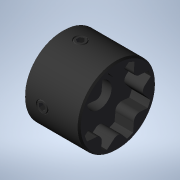
# Autodesk Inventor part: MSF-25 - 6-8 Casing 2
Saved by Autodesk Inventor 2021 (Build 250183000, 183)
## iProperties
Created: 2026-05-20
Part Number: MSF-25 - 6-8 Casing 2
Material: Generic
Catalog Web Link: www.3dfindit.com
Description: MSF right-MSF
Vendor: NBK
Document SubType Name: Modeling
Designer: psAdmin
Manufacturer: NBK
Mass: 6.39983 g
Surface Area: 31.7975 cm^2
Volume: 6.39983 cm^3
Density: 1 g/cm^3
Appearance: PSOLRGB-176-176-176
Category: PARTsolutions
Company: NBK
Title: MSF-25
Author: Cadenas PARTsolutions
Comments: MSF
PSOL_IDENT_0: {$CADENAS_DATA/23d-libs/nbk/motion_control_parts/couplicon_mini/msf/msf_right.prj},174 {VTYP=3D},{NB=
PSOL_IDENT_1: MSF-25 - 6-8 Casing 2},{LINA=MSF-25},{NN=MSF right},{DATE=08.05.2026 02:12:20},{GEOMDATE=08.12.2014
PSOL_IDENT_2: 08:17:09},{VERSION=},{LINEID=40},{WBVAR=D1D2},{WBNUMERIC=}  {NB=MSF-25 - 6-8 Casing 2},{LINA=MSF-25}
PSOL_IDENT_3: ,{KT=DUMMY},{CN=MSF-25},{D1D2=6-8},{D1D2X='6-6','6-6.35','6-8','6-10','6-12','6.35-6.35','6.35-8','6
PSOL_IDENT_4: .35-10','6.35-12','8-8','8-10','8-12','10-10','10-12','12-12'},{A=25},{B=18},{L=12},{W=41},{F=6},{M=
PSOL_IDENT_5: M4},{WT=1.7},{C=17},{K=22},{D=10/10},{NDM=4.000},{KDM=3.242222},{P=0.700},{D1=6},{D2=8},{K1=3.760},{
PSOL_IDENT_6: DU=16.250},{BL=6.000},{H=2.000},{T=1.500}
NB: MSF-25 - 6-8 Casing 2
NN: MSF right
NT: MSF
NBSYN: $CN. - $D1D2. Casing 2
LINA: MSF-25
CATALOG: NBK (Nabeya Bi-tech Kaisha
CN: MSF-25
D1D2: 6-8
D1D2X: '6-6','6-6.35','6-8','6-10','6-12','6.35-6.35','6.35-8','6.35-10','6.35-12','8-8','8-10','8-12','10-10','10-12','12-12'
A: 25
B: 18
L: 12
W: 41
F: 6
M: M4
WT: 1.7
C: 17
K: 22
D: 10/10
NDM: 4
P: 0.7
K1: 3.76
DU: 16.25
BL: 6
H: 2
T: 1.5
SUPPLIER: NBK
ARTICLENO: MSF-25 - 6-8 Casing 2
BOMINFO: MSF-25
CREATOR: CADENAS GmbH
Autodesk Inventor part; units mm, degrees
sketch "Sketch_1" plane through (0, 0, 0) normal (0, 0, 1) x (1, 0, 0)
  line L0 (18, 0) -> (0, 0)
  line L1 (0, 0) -> (0, 12)
  line L2 (0, 12) -> (0.5, 12.5)
  line L3 (0.5, 12.5) -> (17.5, 12.5)
  line L4 (17.5, 12.5) -> (18, 12)
  line L5 (18, 12) -> (18, 0)
  line L6 (18, 0) -> (0, 0)
  constraints: 14 end point
revolve "Revolution1" add sketch "Sketch_1" angle 360 about axis through (18, 0, 0) along (1, 0, 0)
sketch "Sketch_2" plane through (12, 0, 0) normal (1, 0, 0) x (0, 0, -1)
  arc A0 (-10.681, -3.0208) -> (-9.9306, -4.9592) centre (0, 0) ccw
  line L0 (-9.9306, -4.9592) -> (-7.1956, -5.1985)
  arc A1 (-5.1985, -7.1956) -> (-7.1956, -5.1985) centre (-7.0746, -7.0746) ccw
  line L1 (-5.1985, -7.1956) -> (-5.4166, -9.6887)
  arc A2 (-5.4166, -9.6887) -> (-3.5153, -10.5287) centre (0, 0) ccw
  line L2 (-3.5153, -10.5287) -> (-1.4122, -8.764)
  arc A3 (1.4122, -8.764) -> (-1.4122, -8.764) centre (0, -10.005) ccw
  line L3 (1.4122, -8.764) -> (3.0208, -10.681)
  arc A4 (3.0208, -10.681) -> (4.9592, -9.9306) centre (0, 0) ccw
  line L4 (4.9592, -9.9306) -> (5.1985, -7.1956)
  arc A5 (7.1956, -5.1985) -> (5.1985, -7.1956) centre (7.0746, -7.0746) ccw
  line L5 (7.1956, -5.1985) -> (9.6887, -5.4166)
  arc A6 (9.6887, -5.4166) -> (10.5287, -3.5153) centre (0, 0) ccw
  line L6 (10.5287, -3.5153) -> (8.764, -1.4122)
  arc A7 (8.764, 1.4122) -> (8.764, -1.4122) centre (10.005, 0) ccw
  line L7 (8.764, 1.4122) -> (10.681, 3.0208)
  arc A8 (10.681, 3.0208) -> (9.9306, 4.9592) centre (0, 0) ccw
  line L8 (9.9306, 4.9592) -> (7.1956, 5.1985)
  arc A9 (5.1985, 7.1956) -> (7.1956, 5.1985) centre (7.0746, 7.0746) ccw
  line L9 (5.1985, 7.1956) -> (5.4166, 9.6887)
  arc A10 (5.4166, 9.6887) -> (3.5153, 10.5287) centre (0, 0) ccw
  line L10 (3.5153, 10.5287) -> (1.4122, 8.764)
  arc A11 (-1.4122, 8.764) -> (1.4122, 8.764) centre (0, 10.005) ccw
  line L11 (-1.4122, 8.764) -> (-3.0208, 10.681)
  arc A12 (-3.0208, 10.681) -> (-4.9592, 9.9306) centre (0, 0) ccw
  line L12 (-4.9592, 9.9306) -> (-5.1985, 7.1956)
  arc A13 (-7.1956, 5.1985) -> (-5.1985, 7.1956) centre (-7.0746, 7.0746) ccw
  line L13 (-7.1956, 5.1985) -> (-9.6887, 5.4166)
  arc A14 (-9.6887, 5.4166) -> (-10.5287, 3.5153) centre (0, 0) ccw
  line L14 (-10.5287, 3.5153) -> (-8.764, 1.4122)
  arc A15 (-8.764, -1.4122) -> (-8.764, 1.4122) centre (-10.005, 0) ccw
  line L15 (-8.764, -1.4122) -> (-10.681, -3.0208)
  constraints: 32 end point, 32 point on circle, 16 centre point
extrude "Extrusion1" cut sketch "Sketch_2" along normal blind 6
sketch "Sketch3" plane through (0, 0, 0) normal (-1, 0, 0) x (0, 0, 1)
  point P0 (0, 0)
hole "Hole1" at (0, 0, 0) direction (1, 0, 0) diameter 8 depth 12
sketch "Sketch_4" plane through (0, 0, 0) normal (0, 0, 1) x (1, 0, 0)
  line L0 (6, 0) -> (6, 12.5)
  line L1 (6, 12.5) -> (8, 12.5)
  line L2 (8, 12.5) -> (7.6211, 12.1211)
  line L3 (7.6211, 12.1211) -> (7.6211, 0.3789)
  line L4 (7.6211, 0.3789) -> (8, 0)
  line L5 (8, 0) -> (6, 0)
  line L6 (6, 0) -> (6, 12.5)
  constraints: 14 end point
revolve "Revolution2" cut sketch "Sketch_4" angle 360 about axis through (6, 0, 0) along (0, -1, 0)
sketch "Sketch_6" plane through (0, 0, 0) normal (0, 1, 0) x (-1, 0, 0)
  line L0 (-6, 12.5) -> (-6, 0)
  line L1 (-6, 0) -> (-8, 0)
  line L2 (-8, 0) -> (-7.6211, 0.3789)
  line L3 (-7.6211, 0.3789) -> (-7.6211, 12.1211)
  line L4 (-7.6211, 12.1211) -> (-8, 12.5)
  line L5 (-8, 12.5) -> (-6, 12.5)
  line L6 (-6, 12.5) -> (-6, 0)
  constraints: 14 end point
revolve "Revolution3" cut sketch "Sketch_6" angle 360 about axis through (6, 0, 12.5) along (0, 0, 1)
sketch "Sketch_5" plane through (0, 0, -12.5) normal (0, 0, 1) x (1, 0, 0)
  line L0 (11.62, 1.98) -> (11.62, -1.98)
  line L1 (11.62, -1.98) -> (11.9897, -1.98)
  arc A0 (11.9897, -1.98) -> (12.3697, -1.8049) centre (11.9897, -1.48) ccw
  line L2 (12.3697, -1.8049) -> (14.58, 0.78)
  line L3 (14.58, 0.78) -> (14.58, -1.98)
  line L4 (14.58, -1.98) -> (15.18, -1.98)
  line L5 (15.18, -1.98) -> (15.18, 1.98)
  line L6 (15.18, 1.98) -> (14.8103, 1.98)
  arc A1 (14.8103, 1.98) -> (14.4303, 1.8049) centre (14.8103, 1.48) ccw
  line L7 (14.4303, 1.8049) -> (12.22, -0.78)
  line L8 (12.22, -0.78) -> (12.22, 1.98)
  line L9 (12.22, 1.98) -> (11.62, 1.98)
  constraints: 20 end point, 4 point on circle, 2 centre point
extrude "Extrusion2" cut sketch "Sketch_5" along normal blind 0.75
sketch "Sketch_8" plane through (0, 0, -12.5) normal (0, 0, 1) x (1, 0, 0)
  arc A0 (7.0058, 0.1329) -> (7.6, -1.98) centre (7.6, -0.84) ccw
  line L0 (7.6, -1.98) -> (10.08, -1.98)
  line L1 (10.08, -1.98) -> (10.08, 1.98)
  line L2 (10.08, 1.98) -> (7.9, 1.98)
  arc A1 (7.9, 1.98) -> (7.0058, 0.1329) centre (7.9, 0.84) ccw
  arc A2 (7.9, 1.38) -> (7.9, 0.3) centre (7.9, 0.84) ccw
  line L3 (7.9, 0.3) -> (9.48, 0.3)
  line L4 (9.48, 0.3) -> (9.48, 1.38)
  line L5 (9.48, 1.38) -> (7.9, 1.38)
  arc A3 (7.6, -0.3) -> (7.6, -1.38) centre (7.6, -0.84) ccw
  line L6 (7.6, -1.38) -> (9.48, -1.38)
  line L7 (9.48, -1.38) -> (9.48, -0.3)
  line L8 (9.48, -0.3) -> (7.6, -0.3)
  constraints: 18 end point, 8 point on circle, 4 centre point
extrude "Extrusion3" cut sketch "Sketch_8" along normal blind 0.75
sketch "Sketch_9" plane through (0, 0, -12.5) normal (0, 0, 1) x (1, 0, 0)
  line L0 (2.32, 1.38) -> (3.9648, 0)
  line L1 (3.9648, 0) -> (2.32, -1.38)
  line L2 (2.32, -1.38) -> (2.32, -1.98)
  line L3 (2.32, -1.98) -> (2.7016, -1.98)
  arc A0 (2.7016, -1.98) -> (3.0873, -1.8397) centre (2.7016, -1.38) ccw
  line L4 (3.0873, -1.8397) -> (4.68, -0.5034)
  line L5 (4.68, -0.5034) -> (4.68, -1.98)
  line L6 (4.68, -1.98) -> (5.28, -1.98)
  line L7 (5.28, -1.98) -> (5.28, 1.98)
  line L8 (5.28, 1.98) -> (4.68, 1.98)
  line L9 (4.68, 1.98) -> (4.68, 0.5034)
  line L10 (4.68, 0.5034) -> (3.0873, 1.8397)
  arc A1 (3.0873, 1.8397) -> (2.7016, 1.98) centre (2.7016, 1.38) ccw
  line L11 (2.7016, 1.98) -> (2.32, 1.98)
  line L12 (2.32, 1.98) -> (2.32, 1.38)
  constraints: 26 end point, 4 point on circle, 2 centre point
extrude "Extrusion4" cut sketch "Sketch_9" along normal blind 0.75
sketch "Sketch_10" plane through (0, 0, 0) normal (0, 1, 0) x (-1, 0, 0)
  line L0 (-6, 12.5) -> (-6, 6.5)
  line L1 (-6, 6.5) -> (-7.6211, 6.5)
  line L2 (-7.6211, 6.5) -> (-8, 6.8789)
  line L3 (-8, 6.8789) -> (-8, 12.1211)
  line L4 (-8, 12.1211) -> (-7.6211, 12.5)
  line L5 (-7.6211, 12.5) -> (-6, 12.5)
  line L6 (-6, 12.5) -> (-6, 6.5)
  constraints: 14 end point
revolve "Revolution4" add sketch "Sketch_10" angle 360 about axis through (6, 0, 12.5) along (0, 0, 1)
sketch "Sketch_11" plane through (0, 0, 11) normal (0, 0, 1) x (1, 0, 0)
  line L0 (5, -0.5774) -> (6, -1.1547)
  line L1 (6, -1.1547) -> (7, -0.5774)
  line L2 (7, -0.5774) -> (7, 0.5774)
  line L3 (7, 0.5774) -> (6, 1.1547)
  line L4 (6, 1.1547) -> (5, 0.5774)
  line L5 (5, 0.5774) -> (5, -0.5774)
  constraints: 12 end point
extrude "Extrusion5" cut sketch "Sketch_11" along normal blind 1.5
sketch "Sketch_12" plane through (0, 0, 0) normal (0, 0, 1) x (1, 0, 0)
  line L0 (6, 6.5) -> (6, 12.5)
  line L1 (6, 12.5) -> (7.6211, 12.5)
  line L2 (7.6211, 12.5) -> (8, 12.1211)
  line L3 (8, 12.1211) -> (8, 6.8789)
  line L4 (8, 6.8789) -> (7.6211, 6.5)
  line L5 (7.6211, 6.5) -> (6, 6.5)
  line L6 (6, 6.5) -> (6, 12.5)
  constraints: 14 end point
revolve "Revolution5" add sketch "Sketch_12" angle 360 about axis through (6, 6.5, 0) along (0, -1, 0)
sketch "Sketch_13" plane through (0, 11, 0) normal (0, 1, 0) x (1, 0, 0)
  line L0 (5, -0.5774) -> (6, -1.1547)
  line L1 (6, -1.1547) -> (7, -0.5774)
  line L2 (7, -0.5774) -> (7, 0.5774)
  line L3 (7, 0.5774) -> (6, 1.1547)
  line L4 (6, 1.1547) -> (5, 0.5774)
  line L5 (5, 0.5774) -> (5, -0.5774)
  constraints: 12 end point
extrude "Extrusion6" cut sketch "Sketch_13" along normal blind 1.5
ref_plane "left_XY" through (12, 0, 0) normal (1, 0, 0) x (0, 0, -1)
ref_plane "left_YZ" through (12, 0, 0) normal (0, 0, -1) x (0, 1, 0)
ref_plane "left_ZX" through (12, 0, 0) normal (0, 1, 0) x (1, 0, 0)
body "Solid1"
